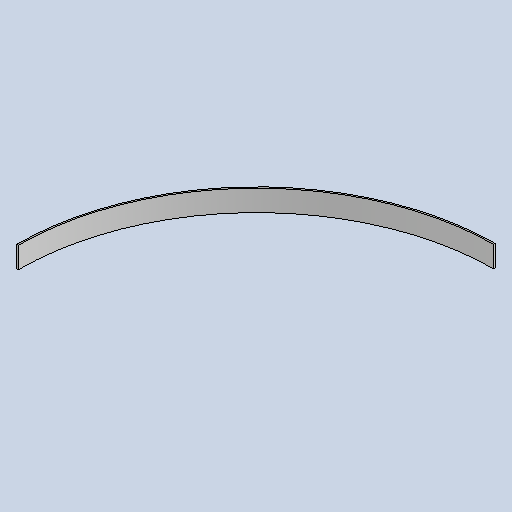
# Autodesk Inventor part: BSH 507 edge amplifier
Saved by Autodesk Inventor 2025 (Build 290162010, 162A)
## iProperties
Created: 2024-09-03
Part Number: BSH 507 edge amplifier
Material: Stainless Steel
Document SubType Name: Sheet Metal
Designer: user
Density: 8 g/cm^3
Sheet Metal Rule: AISI304 3mm Die 32
Sheet Metal Width: 40,000 mm
Sheet Metal Length: 705,923 mm
Sheet Metal Area: 28236,919 mm^2
Appearance: Default
Mass: 677.956 g
Surface Area: 609.736 cm^2
Volume: 84.7445 cm^3
Flat Pattern Width: 4 cm
Flat Pattern Length: 70.5923 cm
Flat Pattern Area: 282.369 cm^2
Author: pokla
Autodesk Inventor part; units mm, degrees
note: some values were not read from the file. Chosen so that the rebuilt part matches the saved one: flange form of "Plate2".
ref_plane "YZ Plane" through (0, 0, 0) normal (1, 0, 0) x (0, 1, 0)
ref_plane "XZ Plane" through (0, 0, 0) normal (0, 1, 0) x (-1, 0, 0)
ref_plane "XY Plane" through (0, 0, 0) normal (0, 0, 1) x (1, 0, 0)
sketch "Sketch3" plane through (0, 0, 0) normal (0, 0, 1) x (1, 0, 0)
  arc A0 (-450, 0) -> (0, 450) centre (0, 0) ccw construction
  line L0 (-450, 0) -> (0, 0) construction
  line L1 (0, 0) -> (0, 450) construction
  arc A1 (0, 450) -> (-3, 449.99) centre (0, 0) ccw construction
  line L2 (0, 0) -> (-3, 449.99) construction
  arc A2 (-3, 449.99) -> (-450, 0) centre (0, 0) ccw
  dimension "d13" = 900
  dimension "d26" = 3
  measures "d13" diameter of A0
  measures "d26" distance of L1.end L2.end
contour flange "Contour Flange1" sketch "Sketch3" thickness 3 bend radius 5 width 40 along (0, 0, 1) mid plane no both sides no wall seen from (-319.2569, 317.1356, 0) lies toward (-0.7094599, 0.7047458, 0) curves A2
bend "Bend1"
corner "Corner1"
equation "\"d14\" = Thickness"
equation "\"d15\" = BendReliefWidth"
equation "\"d16\" = BendReliefDepth"
equation "\"d17\" = MinimumRemnant"
equation "\"d18\" = TransitionRadius"
equation "\"d20\" = BendRadius"
equation "\"d22\" = CornerReliefSize"
equation "\"d23\" = GapSize"
equation "\"d24\" = JacobiRadiusSize"
equation "\"BendReliefWidth\" = Thickness"
equation "\"BendReliefDepth\" = 0.5 * Thickness"
equation "\"CornerReliefSize\" = 4 * Thickness"
equation "\"MinimumRemnant\" = 2 * Thickness"
equation "\"TransitionRadius\" = BendRadius"
equation "\"JacobiRadiusSize\" = BendRadius"
equation "\"GapSize\" = Thickness"
equation "\"Thickness\" = 3"
equation "\"BendRadius\" = 5"
body "Solid2"
